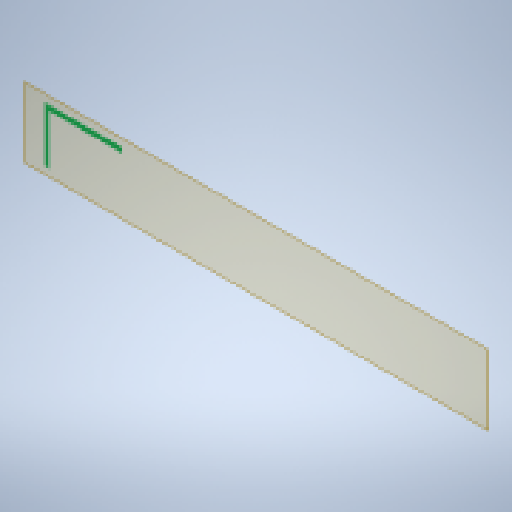
# Autodesk Inventor part: лист
Saved by Autodesk Inventor 2024.2 (Build 282272000, 272)
## iProperties
Created: 2026-02-01
Part Number: лист
Material: Типовые
Document SubType Name: Modeling
Designer: katya_notebook
Density: 1 g/cm^3
Appearance: По умолчанию
Author: katya_notebook
Autodesk Inventor part; units mm, degrees
ref_plane "YZ Plane" through (0, 0, 0) normal (1, 0, 0) x (0, 1, 0)
ref_plane "XZ Plane" through (0, 0, 0) normal (0, 1, 0) x (-1, 0, 0)
ref_plane "XY Plane" through (0, 0, 0) normal (0, 0, 1) x (1, 0, 0)
ref_plane "РабПлоскость1" through (0, 0, 0) normal (0, 0, 1) x (1, 0, 0)
sketch "Эскиз1" plane through (0, 0, 0) normal (0, 0, 1) x (1, 0, 0)
  line L0 (-806.0157, 105) -> (-804.3778, 105) projected
  line L1 (-804.3778, -105) -> (-806.0157, -105) projected
  line L2 (-806.0157, 105) -> (-806.0157, -105)
  line L3 (-806.0157, 105) -> (-509.0157, 105)
  line L4 (-509.0157, 105) -> (-509.0157, -105)
  line L5 (-509.0157, -105) -> (-806.0157, -105)
  line L6 (-786.0157, 85) -> (-509.0157, 85)
  line L7 (-786.0157, 85) -> (-786.0157, -105)
  point P0 (0, 0)
  dimension "d0" = 297
  dimension "d1" = 20
  dimension "d2" = 20
  constraints: 12 end point, 3 perpendicular, 2 point on line, 2 vertical, 1 horizontal
  measures "d0" distance of L0.start L3.end
  measures "d1" distance between parallel lines of L3 L6
  measures "d2" distance between parallel lines of L2 L7
extrude "Выдавливание1" add sketch "Эскиз1" along normal blind 1 contours L0 L3 L4 L6 L7 L5 L1 L2
